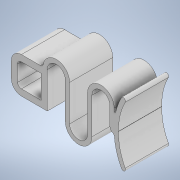
# Autodesk Inventor part: resortePlano1.2mm
Saved by Autodesk Inventor 2021.5 (Build 255421000, 421)
## iProperties
Created: 2024-11-30
Part Number: resortePlano1.2mm
Material: Genérico
Document SubType Name: Modeling
Designer: Joho_
Density: 1 g/cm^3
Appearance: Valor por defecto
Author: Joho_
Autodesk Inventor part; units mm, degrees
ref_plane "YZ Plane" through (0, 0, 0) normal (1, 0, 0) x (0, 1, 0)
ref_plane "XZ Plane" through (0, 0, 0) normal (0, 1, 0) x (-1, 0, 0)
ref_plane "XY Plane" through (0, 0, 0) normal (0, 0, 1) x (1, 0, 0)
sketch "Boceto1" plane through (0, 0, 0) normal (0, 0, 1) x (1, 0, 0)
  line L0 (3, -11.4) -> (3, -5.5)
  line L1 (3, -5.5) -> (-2.2, -5.5)
  arc A0 (-5.5, -2.2) -> (-2.2, -5.5) centre (-2.2, -2.2) ccw
  line L2 (-5.5, -2.2) -> (-5.5, 2.2)
  arc A1 (-2.2, 5.5) -> (-5.5, 2.2) centre (-2.2, 2.2) ccw
  line L3 (-2.2, 5.5) -> (3, 5.5)
  line L4 (3, 5.5) -> (3, 11.4)
  line L5 (3, 3) -> (-2.2, 3)
  arc A2 (-2.2, 3) -> (-3, 2.2) centre (-2.2, 2.2) ccw
  line L6 (-3, 2.2) -> (-3, -2.2)
  arc A3 (-3, -2.2) -> (-2.2, -3) centre (-2.2, -2.2) ccw
  line L7 (-2.2, -3) -> (3, -3)
  line L8 (3, -3) -> (3, 3)
  line L9 (-2.2, 3.25) -> (3.25, 3.25)
  line L10 (3.25, 3.25) -> (3.25, -3.25)
  line L11 (3.25, -3.25) -> (-2.2, -3.25)
  arc A4 (-3.25, -2.2) -> (-2.2, -3.25) centre (-2.2, -2.2) ccw
  line L12 (-3.25, -2.2) -> (-3.25, 2.2)
  arc A5 (-2.2, 3.25) -> (-3.25, 2.2) centre (-2.2, 2.2) ccw
  line L13 (-2.2, 5) -> (5, 5)
  line L14 (5, 5) -> (5, -5)
  line L15 (5, -5) -> (-2.2, -5)
  arc A6 (-5, -2.2) -> (-2.2, -5) centre (-2.2, -2.2) ccw
  line L16 (-5, -2.2) -> (-5, 2.2)
  arc A7 (-2.2, 5) -> (-5, 2.2) centre (-2.2, 2.2) ccw
  line L17 (5, 5) -> (7.5, 5)
  line L18 (10, 5) -> (11.2, 5)
  line L19 (11.2, 5) -> (11.2, -5)
  line L20 (11.2, -5) -> (10, -5)
  line L21 (10, -5) -> (10, 5)
  line L22 (11.2, -5) -> (13.7, -5)
  line L23 (16.2, -5) -> (17.4, -5)
  line L24 (17.4, -5) -> (17.4, 5)
  line L25 (17.4, 5) -> (16.2, 5)
  line L26 (16.2, 5) -> (16.2, -5)
  line L27 (17.4, 5) -> (19.9, 5)
  line L28 (22.4, 5) -> (23.6, 5)
  line L29 (23.6, 5) -> (23.6, 0)
  line L30 (23.6, 0) -> (22.4, 0)
  line L31 (22.4, 0) -> (22.4, 5)
  arc A8 (11.2, 5) -> (3.8, 5) centre (7.5, 5) ccw
  arc A9 (10, 5) -> (5, 5) centre (7.5, 5) ccw
  arc A10 (10, -5) -> (17.4, -5) centre (13.7, -5) ccw
  arc A11 (11.2, -5) -> (16.2, -5) centre (13.7, -5) ccw
  arc A12 (22.4, 5) -> (17.4, 5) centre (19.9, 5) ccw
  arc A13 (23.6, 5) -> (16.2, 5) centre (19.9, 5) ccw
  arc A14 (25.6, 8.5) -> (23.6, 0) centre (40.821, 0.4333) ccw
  circle A15 centre (23.6, 0) radius 1.2
  arc A16 (26.6603, 7.9381) -> (24.7996, 0.0302) centre (40.821, 0.4333) ccw
  line L32 (25.6, 8.5) -> (25.9736, 8.302)
  arc A17 (26.6603, 7.9381) -> (25.6, 8.5) centre (26.1301, 8.219) ccw
  arc A18 (23.6, 0) -> (25.6, -8.5) centre (40.821, -0.4333) ccw
  arc A19 (24.7996, -0.0302) -> (26.6603, -7.9381) centre (40.821, -0.4333) ccw
  line L33 (25.9736, -8.302) -> (26.6603, -7.9381)
  arc A20 (25.6, -8.5) -> (26.6603, -7.9381) centre (26.1301, -8.219) ccw
  point P0 (0, 0)
  point P1 (5, -5)
  point P2 (4.2, -5)
  point P3 (23, 0)
  point P4 (23.6, 1.2)
  point P5 (23.6116, -1.1999)
  point P6 (24.7996, 0.0302)
  point P7 (23.6116, 1.1999)
  dimension "d1" = 0.25
  dimension "d2" = 2
  dimension "d31" = 2.5
  dimension "d33" = 10
  dimension "d34" = 2.5
  dimension "d35" = 1.2
  dimension "d36" = 10
  dimension "d37" = 2.5
  dimension "d41" = 1.2
  constraints: 68 end point, 42 point on circle, 23 centre point, 6 coincident, 6 horizontal, 6 parallel, 3 perpendicular, 3 point on line, 3 other
  measures "d1" distance between parallel lines of L5 L9
  measures "d2" distance between parallel lines of L5 L13
  measures "d31" distance of L13.end L17.end
  measures "d33" distance of L18.end L19.end
  measures "d34" distance of L19.end L22.end
  measures "d35" distance of L25.end L24.end
  measures "d36" distance of L24.end L23.end
  measures "d37" distance of L24.end L27.end
  measures "d41" radial gap between concentric circles of A14 A16
extrude "Extrusión1" add sketch "Boceto1" along normal blind 12 contours L13 L14 L15 A6 L16 A7 | A8 L18 A9 L13 | L19 L20 L21 L18 | A11 L23 A10 L20 | L26 L25 L24 L23 | A13 L28 A12 L25 | L29 A15 L31 L28 | A15 A14 L29 | L29 A14 L30 A15 | L30 A18 A15 | A14 A15 A18 L29 | L29 A14 | A14 A17 A16 A15 | A15 A19 A20 A18
fillet "Empalme1" radius 0.8 2 edges at (3.8, 5, 6) (23.6116, -1.1999, 6)
fillet "Empalme1" radius 0.2 2 edges at (23.6, 1.2, 6) (23.6116, 1.1999, 6)
